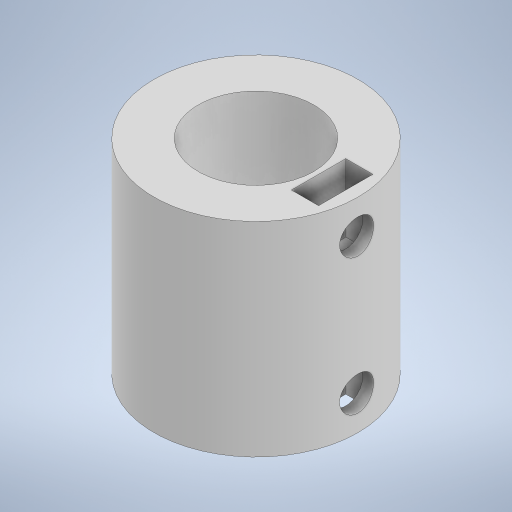
# Autodesk Inventor part: collar
Saved by Autodesk Inventor 2023 (Build 270158000, 158)
## iProperties
Created: 2022-11-01
Part Number: collar
Material: Generic
Document SubType Name: Modeling
Designer: neera
Density: 1 g/cm^3
Appearance: Default
Author: neera
Autodesk Inventor part; units mm, degrees
ref_plane "YZ Plane" through (0, 0, 0) normal (1, 0, 0) x (0, 1, 0)
ref_plane "XZ Plane" through (0, 0, 0) normal (0, 1, 0) x (-1, 0, 0)
ref_plane "XY Plane" through (0, 0, 0) normal (0, 0, 1) x (1, 0, 0)
sketch "Sketch1" plane through (0, 0, 0) normal (0, 1, 0) x (-1, 0, 0)
  circle A0 centre (0, 0) radius 7.5
  arc A1 (-2.6551, -1.695) -> (-2.6551, 1.695) centre (0, 0) ccw
  line L0 (-2.6551, 1.695) -> (-2.6551, -1.695)
  dimension "d0" = 15
  dimension "d1" = 6.3
  dimension "d8" = 3.39
  constraints: 2 centre point, 2 coincident, 2 end point, 2 point on circle, 1 vertical
  measures "d0" diameter of A0
  measures "d1" diameter of A1
  measures "d8" distance of L0.start L0.end
extrude "Extrusion2" add sketch "Sketch1" along normal blind 15
sketch "Sketch3" plane through (0, 15, 0) normal (0, 1, 0) x (1, 0, 0)
  circle A0 centre (0, 0) radius 4.25
  dimension "d11" = 8.5
  constraints: 1 centre point, 1 coincident
  measures "d11" diameter of A0
extrude "Extrusion3" cut sketch "Sketch3" against normal blind 7.5
sketch "Sketch4" plane through (0, 15, 0) normal (0, 1, 0) x (1, 0, 0)
  line L0 (6.6, 2) -> (4.6, 2)
  line L1 (4.6, 2) -> (4.6, -2)
  line L2 (4.6, -2) -> (6.6, -2)
  line L3 (6.6, -2) -> (6.6, 2)
  circle A0 centre (0, 0) radius 4.25 projected
  point P0 (5.6, 2)
  dimension "d14" = 2
  dimension "d15" = 4
  dimension "d16" = 2
  dimension "d17" = 4.6
  constraints: 8 end point, 2 parallel, 1 horizontal, 1 midpoint, 1 perpendicular
  measures "d14" distance of L2.end L1.end
  measures "d15" distance of L1.end L0.end
  measures "d16" vertical distance of point (0, 0) point (5.6, 2)
  measures "d17" distance from line of A0.centre L1
extrude "Extrusion4" cut sketch "Sketch4" against normal blind 5 contours L3 L2 L1 L0
sketch "Sketch5" plane through (0, 0, 0) normal (0, -1, 0) x (1, 0, 0)
  line L0 (6.6, 2) -> (4.6, 2) projected
  line L1 (4.6, -2) -> (6.6, -2) projected
  line L2 (6.6, 2) -> (4.6, 2)
  line L3 (4.6, 2) -> (4.6, -2)
  line L4 (4.6, -2) -> (6.6, -2)
  line L5 (6.6, -2) -> (6.6, 2)
  point P0 (0, 0)
  point P1 (4.6, 2)
  point P2 (6.6, -2)
  constraints: 8 end point, 2 parallel, 1 horizontal, 1 perpendicular
extrude "Extrusion5" cut sketch "Sketch5" against normal blind 5
sketch "Sketch6" plane through (4.6, 15, 2) normal (1, 0, 0) x (0, 0, -1)
  circle A0 centre (2, -2.5) radius 1.25
  line L0 (4, 0) -> (4, -5) projected
  line L1 (4, -5) -> (0, -5) projected
  circle A1 centre (2, -12.5) radius 1.25
  line L2 (3.695, -15) -> (3.695, -7.5) projected
  line L3 (4, -15) -> (4, -10) projected
  line L4 (9.5, -15) -> (-5.5, -15) projected
  point P0 (2, -15)
  dimension "d22" = 2.5
  dimension "d23" = 2
  dimension "d24" = 2.5
  dimension "d25" = 2.5
  dimension "d27" = 2
  dimension "d28" = 2.5
  constraints: 2 centre point
  measures "d22" diameter of A0
  measures "d23" distance from line of L0 A0.centre
  measures "d24" distance from line of A0.centre L1
  measures "d25" diameter of A1
  measures "d27" distance from line of L3 A1.centre
  measures "d28" distance from line of L4 A1.centre
extrude "Extrusion6" cut sketch "Sketch6" along normal blind 5
body "Solid2"
